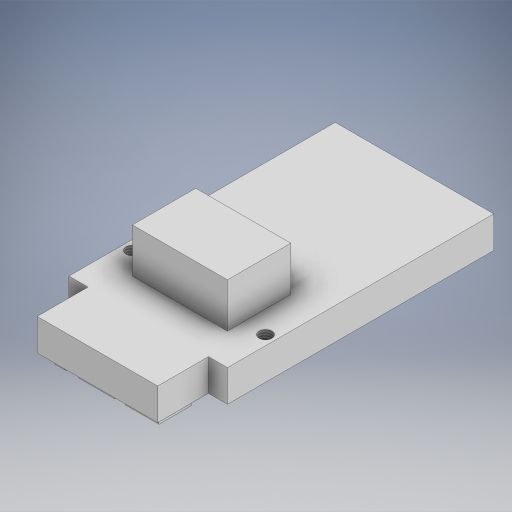
# Autodesk Inventor part: Head
Saved by Autodesk Inventor 2023 (Build 270158000, 158)
## iProperties
Created: 2024-04-01
Part Number: Head
Material: Generic
Document SubType Name: Modeling
Designer: andrew
Density: 1 g/cm^3
Appearance: Default
Author: andrew
Autodesk Inventor part; units mm, degrees
ref_plane "YZ Plane" through (0, 0, 0) normal (1, 0, 0) x (0, 1, 0)
ref_plane "XZ Plane" through (0, 0, 0) normal (0, 1, 0) x (-1, 0, 0)
ref_plane "XY Plane" through (0, 0, 0) normal (0, 0, 1) x (1, 0, 0)
sketch "Sketch1" plane through (0, 0, 0) normal (0, 1, 0) x (-1, 0, 0)
  line L0 (0, 0) -> (25, 0)
  line L1 (25, 0) -> (25, -42)
  line L2 (25, -42) -> (0, -42)
  line L3 (0, -42) -> (0, 0)
  line L4 (22, 0) -> (3, 0)
  line L5 (3, 0) -> (3, 8)
  line L6 (3, 8) -> (22, 8)
  line L7 (22, 8) -> (22, 0)
  point P0 (22, 4)
  dimension "d0" = 19
  dimension "d1" = 3
  dimension "d2" = 3
  dimension "d3" = 42
  dimension "d4" = 25
  dimension "d27" = 8
  constraints: 16 end point, 4 parallel, 2 horizontal, 2 perpendicular, 1 midpoint, 1 point on line
  measures "d0" distance of L5.end L6.end
  measures "d1" distance between parallel lines of L3 L5
  measures "d2" distance from line of point (22, 4) L1
  measures "d3" distance of L0.end L1.end
  measures "d4" distance of L1.end L2.end
  measures "d27" distance of L4.end L5.end
extrude "Extrusion1" add sketch "Sketch1" along normal blind 5
sketch "Sketch2" plane through (0, 5, 0) normal (0, 1, 0) x (1, 0, 0)
  line L0 (-20, 5) -> (-5, 5)
  line L1 (-5, 5) -> (-5, 15)
  line L2 (-5, 15) -> (-20, 15)
  line L3 (-20, 15) -> (-20, 5)
  line L4 (-25, 0) -> (-22, 0) projected
  line L5 (-25, 42) -> (-25, 0) projected
  line L6 (0, 0) -> (0, 42) projected
  dimension "d7" = 5
  dimension "d8" = 10
  dimension "d25" = 5
  dimension "d26" = 5
  constraints: 8 end point, 2 parallel, 1 horizontal, 1 perpendicular
  measures "d7" distance between parallel lines of L4 L0
  measures "d8" distance of L2.end L0.start
  measures "d25" distance between parallel lines of L5 L3
  measures "d26" distance between parallel lines of L6 L1
extrude "Extrusion2" add sketch "Sketch2" along normal blind 7
sketch "Sketch3" plane through (0, 0, 0) normal (0, -1, 0) x (1, 0, 0)
  circle A0 centre (-1.5, -7.5) radius 1
  line L0 (-3, 0) -> (0, 0) projected
  line L1 (0, 0) -> (0, -42) projected
  circle A1 centre (-23.5, -8.5) radius 1
  line L2 (-25, 0) -> (-22, 0) projected
  line L3 (-25, -42) -> (-25, 0) projected
  dimension "d13" = 2
  dimension "d14" = 7.5
  dimension "d15" = 1.5
  dimension "d16" = 2
  dimension "d17" = 8.5
  dimension "d18" = 1.5
  constraints: 2 centre point
  measures "d13" diameter of A0
  measures "d14" distance from line of L0 A0.centre
  measures "d15" distance from line of L1 A0.centre
  measures "d16" diameter of A1
  measures "d17" distance from line of L2 A1.centre
  measures "d18" distance from line of L3 A1.centre
extrude "Extrusion3" cut sketch "Sketch3" against normal blind 7
thread "Thread1" size "M2x0.4" class "6H" standard "ANSI Metric M Profile" full length
thread "Thread2" size "M2x0.4" class "6H" standard "ANSI Metric M Profile" full length
sketch "Sketch4" plane through (0, 0, 0) normal (0, -1, 0) x (1, 0, 0)
  line L0 (-3.66, 7.1394) -> (-3.66, 2.0183)
  line L1 (-3.66, 2.0183) -> (-7.1475, 2.0183)
  line L2 (-7.1475, 5.8905) -> (-7.1475, 7.1394)
  line L3 (-7.1475, 7.1394) -> (-3.66, 7.1394)
  line L4 (-7.1475, 5.8905) -> (-8.5429, 2.0183)
  line L5 (-8.5429, 2.0183) -> (-10.2962, 2.0183)
  line L6 (-10.2962, 2.0183) -> (-12.2596, 4.8754)
  line L7 (-12.2596, 4.8754) -> (-12.2596, 7.1394)
  line L8 (-12.2596, 7.1394) -> (-10.6175, 7.1394)
  line L9 (-10.6175, 7.1394) -> (-10.6175, 4.8754)
  line L10 (-10.6175, 4.8754) -> (-8.9607, 4.8754)
  line L11 (-8.9607, 4.8754) -> (-8.9607, 7.1394)
  line L12 (-8.9607, 7.1394) -> (-7.1475, 7.1394)
  line L13 (-12.2596, 4.8754) -> (-12.2596, 2.0183)
  line L14 (-14.9412, 1.77) -> (-14.9412, 3.503)
  line L15 (-13.1457, 3.503) -> (-13.1457, 6.1648)
  line L16 (-13.1457, 6.1648) -> (-14.9412, 6.1648)
  line L17 (-14.9412, 6.1648) -> (-14.9412, 7.1394)
  line L18 (-12.2596, 7.1394) -> (-14.9412, 7.1394)
  line L19 (-12.2596, 2.0183) -> (-12.2596, 1.8295)
  line L20 (-14.9412, 3.503) -> (-14.9412, 6.1648)
  line L21 (-7.1475, 2.0183) -> (-7.1475, 4.4084)
  line L22 (-7.1475, 4.4084) -> (-4.6775, 4.4084)
  line L23 (-4.6775, 4.4084) -> (-4.6775, 5.2007)
  line L24 (-4.6775, 5.2007) -> (-7.1475, 5.2007)
  line L25 (-7.1475, 5.2007) -> (-7.1475, 5.8905)
  line L26 (-4.6775, 3.503) -> (-4.6775, 2.6365)
  line L27 (-4.6775, 2.6365) -> (-6.5324, 2.6365)
  line L28 (-6.5324, 2.6365) -> (-6.5324, 3.503)
  line L29 (-6.5324, 3.503) -> (-4.6775, 3.503)
  line L30 (-4.66, 5.8905) -> (-6.5324, 5.8905)
  line L31 (-6.5324, 5.8905) -> (-6.5324, 6.7449)
  line L32 (-6.5324, 6.7449) -> (-4.9174, 6.7449)
  line L33 (-4.9174, 6.7449) -> (-4.66, 5.8905)
  line L34 (-14.9412, 1.77) -> (-16.3182, 1.77)
  line L35 (-16.3182, 1.77) -> (-16.3182, 7.1394)
  line L36 (-16.3182, 7.1394) -> (-14.9412, 7.1394)
  line L37 (-18.5068, 5.8905) -> (-16.4834, 4.2767)
  line L38 (-16.4834, 4.2767) -> (-19.3704, 1.77)
  line L39 (-19.3704, 1.77) -> (-17.9269, 1.77)
  line L40 (-17.9269, 1.77) -> (-16.3182, 3.1668)
  line L41 (-18.5068, 5.8905) -> (-20.0727, 7.1394)
  line L42 (-20.0727, 7.1394) -> (-18.5068, 7.1394)
  line L43 (-16.3182, 5.8905) -> (-18.5068, 7.1394)
  line L44 (-9.0583, 2.869) -> (-10.6175, 2.869)
  line L45 (-10.6175, 2.869) -> (-10.6175, 3.7284)
  line L46 (-10.6175, 3.7284) -> (-9.0583, 3.7284)
  line L47 (-9.0583, 3.7284) -> (-9.0583, 2.869)
  line L48 (-14.0417, 3.5591) -> (-14.15, 1.8295)
  line L49 (-12.2596, 1.8295) -> (-14.15, 1.8295)
  line L50 (-14.0452, 3.503) -> (-13.1457, 3.503)
  line L51 (-2.7778, -34.9531) -> (-2.7778, -41.136)
  line L52 (-2.7778, -41.136) -> (-8.4213, -41.136)
  line L53 (-8.4213, -41.136) -> (-8.4213, -39.4983)
  line L54 (-8.4213, -39.4983) -> (-4.4166, -39.4983)
  line L55 (-4.4166, -39.4983) -> (-4.4166, -38.0343)
  line L56 (-4.4166, -38.0343) -> (-9.0583, -38.0343)
  line L57 (-9.0583, -38.0343) -> (-8.4213, -36.2667)
  line L58 (-8.4213, -36.2667) -> (-4.4166, -36.2667)
  line L59 (-4.4166, -36.2667) -> (-4.4166, -33.2701)
  line L60 (-4.4166, -33.2701) -> (-2.3323, -33.7168)
  line L61 (-2.3323, -33.7168) -> (-2.7778, -34.9531)
  line L62 (-10.176, -41.136) -> (-9.8379, -32.7739)
  line L63 (-9.8379, -32.7739) -> (-12.2596, -33.2701)
  line L64 (-12.2596, -33.2701) -> (-11.8606, -36.5207)
  line L65 (-11.8606, -36.5207) -> (-13.5954, -36.9549)
  line L66 (-13.5954, -36.9549) -> (-14.8005, -36.5207)
  line L67 (-14.8005, -36.5207) -> (-15.3476, -34.335)
  line L68 (-15.3476, -34.335) -> (-15.6141, -33.2701)
  line L69 (-15.6141, -33.2701) -> (-16.8071, -32.8402)
  line L70 (-16.8071, -32.8402) -> (-16.8627, -34.2134)
  line L71 (-16.8627, -34.2134) -> (-16.9559, -36.5207)
  line L72 (-16.9559, -36.5207) -> (-16.6555, -37.7209)
  arc A0 (-15.6141, -37.7209) -> (-16.6555, -37.7209) centre (-16.1348, -39.8012) ccw
  line L73 (-15.6141, -37.7209) -> (-14.4216, -38.0343)
  line L74 (-14.4216, -38.0343) -> (-16.3182, -39.1953)
  line L75 (-16.3182, -39.1953) -> (-16.9559, -41.136)
  line L76 (-16.9559, -41.136) -> (-10.176, -41.136)
  circle A1 centre (-13.2048, -39.1953) radius 1.2392
  circle A2 centre (-18.8951, -37.3841) radius 1.5485
  line L77 (-21.1041, -32.8402) -> (-20.4436, -35.3671)
  line L78 (-20.4436, -35.3671) -> (-22.4923, -35.3671)
  line L79 (-22.4923, -35.3671) -> (-22.4923, -32.8402)
  line L80 (-22.4923, -32.8402) -> (-22.059, -32.8402)
  line L81 (-22.059, -32.8402) -> (-22.059, -34.4396)
  line L82 (-22.059, -34.4396) -> (-21.468, -34.4396)
  line L83 (-21.468, -34.4396) -> (-21.1041, -32.8402)
  line L84 (-23.4723, -32.8402) -> (-24.287, -32.8402)
  line L85 (-24.287, -32.8402) -> (-24.287, -39.8012)
  line L86 (-24.287, -39.8012) -> (-24.9664, -39.8012)
  line L87 (-24.9664, -39.8012) -> (-24.538, -41.4401)
  line L88 (-24.538, -41.4401) -> (-17.5177, -41.4401)
  line L89 (-17.5177, -41.4401) -> (-17.9667, -39.7224)
  line L90 (-17.9667, -39.7224) -> (-23.8797, -39.7224)
  line L91 (-23.8797, -39.7224) -> (-23.4723, -32.8402)
  point P0 (0, 0)
  constraints: 184 end point, 36 point on line, 34 perpendicular, 14 parallel, 6 horizontal, 5 vertical, 3 centre point, 2 point on circle
extrude "Extrusion4" add sketch "Sketch4" along normal blind 1
body "Solid1"
